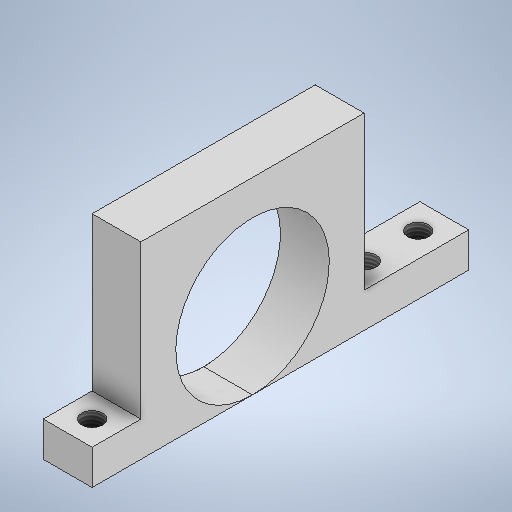
# Autodesk Inventor part: aguanta rolinera
Saved by Autodesk Inventor 2025.2 (Build 292293000, 293)
## iProperties
Created: 2025-03-30
Part Number: aguanta rolinera
Material: Generic
Document SubType Name: Modeling
Designer: maqmat
Density: 1 g/cm^3
Appearance: Default
Author: maqmat
Autodesk Inventor part; units mm, degrees
ref_plane "YZ Plane" through (0, 0, 0) normal (1, 0, 0) x (0, 1, 0)
ref_plane "XZ Plane" through (0, 0, 0) normal (0, 1, 0) x (-1, 0, 0)
ref_plane "XY Plane" through (0, 0, 0) normal (0, 0, 1) x (1, 0, 0)
sketch "Sketch1" plane through (0, 0, 0) normal (1, 0, 0) x (0, 1, 0)
  circle A0 centre (0, 0) radius 11
  line L0 (0, 16) -> (-11, 16)
  line L1 (-11, 16) -> (-11, -16)
  line L2 (-11, -16) -> (11, -16)
  line L3 (11, -16) -> (11, 16)
  line L4 (11, 16) -> (0, 16)
  line L5 (-11, 16) -> (-11, 23)
  line L6 (-11, 23) -> (-6, 23)
  line L7 (-6, 23) -> (-6, 16)
  line L8 (-11, -16) -> (-11, -31)
  line L9 (-11, -31) -> (-6, -31)
  line L10 (-6, -31) -> (-6, -16)
  point P0 (11, 0)
  point P1 (-11, 0)
  dimension "d0" = 22
  dimension "d4" = 7
  dimension "d5" = 5
  dimension "d6" = 15
  constraints: 22 end point, 7 perpendicular, 7 point on line, 1 centre point, 1 coincident
  measures "d0" diameter of A0
  measures "d4" distance of L0.end L5.end
  measures "d5" distance of L5.end L6.end
  measures "d6" distance of L1.end L8.end
extrude "Extrusion1" add sketch "Sketch1" against normal blind 7 contours L3 L2 L1 A0 | A0 L1 L0 L4 L3 | L5 L6 L7 L0 | L2 L10 L9 L8
sketch "Sketch2" plane through (0, 11, 16) normal (0, 1, 0) x (1, 0, 0)
  line L0 (-7, 16) -> (-7, 32) projected
  line L1 (0, 16) -> (0, 0) projected
  line L2 (-7, 32) -> (0, 32)
  line L3 (0, 32) -> (0, 0)
  line L4 (0, 0) -> (-7, 0)
  line L5 (-7, 0) -> (-7, 32)
  constraints: 8 end point, 2 parallel, 1 horizontal, 1 perpendicular
extrude "Extrusion2" add sketch "Sketch2" along normal blind 5
sketch "Sketch3" plane through (0, -6, 23) normal (0, 1, 0) x (1, 0, 0)
  line L0 (0, 7) -> (0, 0) projected
  line L1 (-7, 0) -> (-7, 7) projected
  line L2 (0, 0) -> (-7, 0) projected
  line L3 (0, 7) -> (-7, 7) projected
  circle A0 centre (-3.5, 3.5) radius 1.5
  line L4 (0, 54) -> (0, 39) projected
  line L5 (-7, 39) -> (-7, 54) projected
  line L6 (0, 54) -> (-7, 54) projected
  line L7 (0, 39) -> (-7, 39) projected
  line L8 (0, 46.5) -> (0, 39)
  line L9 (0, 23) -> (0, 54) projected
  line L10 (0, 46.5) -> (0, 54)
  line L11 (0, 54) -> (0, 50.25)
  line L12 (-7, 54) -> (-7, 23) projected
  circle A1 centre (-3.5, 42.75) radius 1.5
  circle A2 centre (-3.5, 50.25) radius 1.5
  dimension "d11" = 3
  dimension "d12" = 3
  constraints: 6 end point, 3 centre point, 2 midpoint, 2 point on line
  measures "d11" diameter of A0
  measures "d12" diameter of A1
extrude "Extrusion3" cut sketch "Sketch3" against normal blind 5 contours A0
extrude "Extrusion4" cut sketch "Sketch3" against normal blind 5 contours A1
extrude "Extrusion5" cut sketch "Sketch3" against normal blind 5 contours A2
thread "Thread1" size "M3x0.5" class "6H" standard "ANSI Metric M Profile" full length
thread "Thread2" size "M3x0.5" class "6H" standard "ANSI Metric M Profile" full length
thread "Thread3" size "M3x0.5" class "6H" standard "ANSI Metric M Profile" full length
body "Solid1"
